Autodesk Inventor part; units mm, degrees
(part 2 of 2)
  spline S23 degree 3 poles (-70.3102, 10.593) (-70.1991, 10.6097) (-69.9769, 10.6432) (-69.6422, 10.6835) (-69.3067, 10.7162) (-68.9704, 10.7401) (-68.6336, 10.7549) (-68.2966, 10.7599) (-67.9595, 10.7543) (-67.6228, 10.7372) (-67.3429, 10.7123) (-67.1199, 10.6849) (-66.9531, 10.6603) (-66.787, 10.6316) (-66.6222, 10.5966) (-66.4851, 10.5659) (-66.3739, 10.5488) (-66.2901, 10.5406) (-66.2059, 10.536) (-66.1216, 10.5362) (-66.0374, 10.5419) (-65.9539, 10.5535) (-65.8715, 10.5716) (-65.7908, 10.5963) (-65.7126, 10.628) (-65.638, 10.6674) (-65.5675, 10.7136) (-65.501, 10.7656) (-65.4412, 10.8252) (-65.3876, 10.8903) (-65.3403, 10.9603) (-65.2902, 11.0611) (-65.2358, 11.1905) (-65.176, 11.3176) (-65.1345, 11.4222) (-65.1141, 11.5042) (-65.1017, 11.5876) (-65.0973, 11.6719) (-65.1031, 11.7561) (-65.1159, 11.8394) (-65.1366, 11.9213) (-65.1653, 12.0006) (-65.2008, 12.0771) (-65.2425, 12.1504) (-65.2898, 12.2203) (-65.3418, 12.2867) (-65.3981, 12.3495) (-65.4578, 12.4089) (-65.52, 12.4658) (-65.607, 12.537) (-65.7215, 12.6184) (-65.8578, 12.7175) (-65.9903, 12.8218) (-66.1201, 12.9293) (-66.2896, 13.0769) (-66.4953, 13.2682) (-66.7333, 13.5071) (-66.9629, 13.7539) (-67.1846, 14.0078) (-67.3988, 14.2681) (-67.606, 14.5341) (-67.8061, 14.8054) (-68, 15.0811) (-68.1237, 15.2687) (-68.1856, 15.3625) knots -1.078574 -1.078574 -1.078574 -1.078574 -1.044867 -1.011159 -0.977452 -0.943745 -0.910038 -0.876331 -0.842624 -0.808918 -0.775212 -0.758359 -0.741505 -0.724651 -0.707798 -0.690947 -0.68252 -0.674093 -0.665668 -0.657242 -0.648815 -0.640389 -0.631963 -0.623537 -0.61511 -0.606685 -0.598264 -0.589839 -0.581413 -0.57299 -0.564565 -0.556141 -0.539287 -0.522433 -0.514009 -0.505584 -0.49716 -0.488735 -0.48031 -0.471889 -0.463464 -0.455037 -0.446611 -0.438185 -0.429758 -0.421332 -0.412906 -0.40448 -0.396053 -0.387627 -0.370775 -0.353922 -0.337069 -0.320215 -0.303361 -0.269656 -0.235949 -0.202243 -0.168536 -0.134829 -0.101122 -0.067415 -0.033707 0 0 0 0 construction
  arc A27 (-67.448, 16.6395) -> (-68.1856, 15.3625) centre (-40.1144, 0) ccw construction
  spline S24 degree 3 poles (-67.448, 16.6395) (-67.3358, 16.6328) (-67.1115, 16.6194) (-66.7757, 16.5892) (-66.4407, 16.5514) (-66.1069, 16.5049) (-65.7744, 16.4494) (-65.4436, 16.3842) (-65.115, 16.3087) (-64.7893, 16.2219) (-64.5207, 16.1393) (-64.3082, 16.0662) (-64.1502, 16.0075) (-63.9937, 15.9448) (-63.8398, 15.8763) (-63.712, 15.8177) (-63.6069, 15.778) (-63.5265, 15.7525) (-63.4452, 15.7305) (-63.3627, 15.7131) (-63.2792, 15.7012) (-63.195, 15.6952) (-63.1107, 15.6957) (-63.0267, 15.7031) (-62.9436, 15.7179) (-62.8624, 15.7409) (-62.7838, 15.7715) (-62.708, 15.8085) (-62.6371, 15.8544) (-62.5711, 15.9069) (-62.5103, 15.9655) (-62.4404, 16.0537) (-62.3602, 16.169) (-62.2753, 16.2809) (-62.213, 16.3746) (-62.176, 16.4505) (-62.1464, 16.5295) (-62.1246, 16.6111) (-62.1128, 16.6946) (-62.108, 16.7788) (-62.1112, 16.8632) (-62.1228, 16.9467) (-62.1417, 17.029) (-62.1672, 17.1094) (-62.1989, 17.1875) (-62.236, 17.2633) (-62.2779, 17.3364) (-62.324, 17.407) (-62.373, 17.4756) (-62.4433, 17.5633) (-62.5384, 17.6667) (-62.6511, 17.792) (-62.759, 17.9215) (-62.8636, 18.0537) (-62.9988, 18.2332) (-63.1602, 18.4632) (-63.3433, 18.7463) (-63.5166, 19.0355) (-63.6806, 19.33) (-63.8361, 19.6291) (-63.9834, 19.9323) (-64.1227, 20.2393) (-64.2551, 20.5493) (-64.3371, 20.7586) (-64.3781, 20.8632) knots -1.078574 -1.078574 -1.078574 -1.078574 -1.044867 -1.011159 -0.977452 -0.943745 -0.910038 -0.876331 -0.842624 -0.808918 -0.775212 -0.758359 -0.741505 -0.724651 -0.707798 -0.690947 -0.68252 -0.674093 -0.665668 -0.657242 -0.648815 -0.640389 -0.631963 -0.623537 -0.61511 -0.606685 -0.598264 -0.589839 -0.581413 -0.57299 -0.564565 -0.556141 -0.539287 -0.522433 -0.514009 -0.505584 -0.49716 -0.488735 -0.48031 -0.471889 -0.463464 -0.455037 -0.446611 -0.438185 -0.429758 -0.421332 -0.412906 -0.40448 -0.396053 -0.387627 -0.370775 -0.353922 -0.337069 -0.320215 -0.303361 -0.269656 -0.235949 -0.202243 -0.168536 -0.134829 -0.101122 -0.067415 -0.033707 0 0 0 0 construction
  arc A28 (-63.3911, 21.9589) -> (-64.3781, 20.8632) centre (-40.1144, 0) ccw construction
  spline S25 degree 3 poles (-63.3911, 21.9589) (-63.2828, 21.929) (-63.0662, 21.8693) (-62.744, 21.7699) (-62.4242, 21.6633) (-62.1073, 21.5484) (-61.7936, 21.4249) (-61.4836, 21.2924) (-61.178, 21.1502) (-60.8773, 20.9976) (-60.6318, 20.861) (-60.4392, 20.7453) (-60.2968, 20.655) (-60.1568, 20.5612) (-60.0204, 20.4621) (-59.9077, 20.3783) (-59.8131, 20.3175) (-59.7398, 20.276) (-59.6648, 20.2375) (-59.5877, 20.2034) (-59.5085, 20.1743) (-59.4275, 20.151) (-59.3448, 20.134) (-59.2611, 20.1237) (-59.1768, 20.1209) (-59.0926, 20.1265) (-59.0093, 20.1401) (-58.9275, 20.1605) (-58.8486, 20.1907) (-58.7731, 20.2283) (-58.7014, 20.273) (-58.6147, 20.3447) (-58.5124, 20.4409) (-58.406, 20.5326) (-58.3256, 20.6113) (-58.2736, 20.6779) (-58.2283, 20.749) (-58.19, 20.8243) (-58.1611, 20.9036) (-58.1389, 20.9849) (-58.1245, 21.0681) (-58.1184, 21.1522) (-58.1198, 21.2366) (-58.1281, 21.3205) (-58.1428, 21.4036) (-58.1633, 21.4854) (-58.1892, 21.5656) (-58.2196, 21.6442) (-58.2532, 21.7215) (-58.3038, 21.8219) (-58.3753, 21.9429) (-58.4595, 22.0889) (-58.5381, 22.238) (-58.6129, 22.389) (-58.7078, 22.5927) (-58.8179, 22.8512) (-58.9381, 23.1662) (-59.0475, 23.4851) (-59.1467, 23.8073) (-59.2366, 24.1322) (-59.3177, 24.4594) (-59.3901, 24.7886) (-59.4551, 25.1194) (-59.4918, 25.3411) (-59.5102, 25.452) knots -1.078574 -1.078574 -1.078574 -1.078574 -1.044867 -1.011159 -0.977452 -0.943745 -0.910038 -0.876331 -0.842624 -0.808918 -0.775212 -0.758359 -0.741505 -0.724651 -0.707798 -0.690947 -0.68252 -0.674093 -0.665668 -0.657242 -0.648815 -0.640389 -0.631963 -0.623537 -0.61511 -0.606685 -0.598264 -0.589839 -0.581413 -0.57299 -0.564565 -0.556141 -0.539287 -0.522433 -0.514009 -0.505584 -0.49716 -0.488735 -0.48031 -0.471889 -0.463464 -0.455037 -0.446611 -0.438185 -0.429758 -0.421332 -0.412906 -0.40448 -0.396053 -0.387627 -0.370775 -0.353922 -0.337069 -0.320215 -0.303361 -0.269656 -0.235949 -0.202243 -0.168536 -0.134829 -0.101122 -0.067415 -0.033707 0 0 0 0 construction
  arc A29 (-58.3169, 26.3186) -> (-59.5102, 25.452) centre (-40.1144, 0) ccw construction
  spline S26 degree 3 poles (-58.3169, 26.3186) (-58.2172, 26.2668) (-58.0177, 26.1633) (-57.7233, 25.9992) (-57.4326, 25.8284) (-57.1465, 25.6501) (-56.8654, 25.4641) (-56.5897, 25.27) (-56.3203, 25.0674) (-56.058, 24.8556) (-55.8462, 24.6709) (-55.6818, 24.5177) (-55.5614, 24.3998) (-55.4439, 24.2789) (-55.3311, 24.1537) (-55.2383, 24.0483) (-55.1584, 23.9691) (-55.0953, 23.9132) (-55.03, 23.86) (-54.9616, 23.8106) (-54.8902, 23.7657) (-54.8158, 23.7261) (-54.7385, 23.6922) (-54.6587, 23.6648) (-54.5768, 23.6445) (-54.4933, 23.6325) (-54.4091, 23.6284) (-54.3247, 23.6314) (-54.2413, 23.6446) (-54.1597, 23.6656) (-54.0803, 23.6945) (-53.9805, 23.7466) (-53.8604, 23.8194) (-53.7373, 23.887) (-53.6423, 23.9472) (-53.5776, 24.0015) (-53.5185, 24.0617) (-53.4654, 24.1273) (-53.4206, 24.1989) (-53.382, 24.2738) (-53.3506, 24.3522) (-53.3272, 24.4332) (-53.311, 24.516) (-53.3016, 24.5999) (-53.2988, 24.6842) (-53.3019, 24.7684) (-53.3105, 24.8523) (-53.3238, 24.9355) (-53.3407, 25.0181) (-53.3692, 25.1269) (-53.414, 25.26) (-53.4661, 25.4203) (-53.5119, 25.5825) (-53.5538, 25.7458) (-53.6042, 25.9648) (-53.6582, 26.2405) (-53.7103, 26.5736) (-53.7509, 26.9083) (-53.781, 27.2441) (-53.8014, 27.5806) (-53.8126, 27.9175) (-53.8151, 28.2546) (-53.8099, 28.5917) (-53.7997, 28.8161) (-53.7946, 28.9284) knots -1.078574 -1.078574 -1.078574 -1.078574 -1.044867 -1.011159 -0.977452 -0.943745 -0.910038 -0.876331 -0.842624 -0.808918 -0.775212 -0.758359 -0.741505 -0.724651 -0.707798 -0.690947 -0.68252 -0.674093 -0.665668 -0.657242 -0.648815 -0.640389 -0.631963 -0.623537 -0.61511 -0.606685 -0.598264 -0.589839 -0.581413 -0.57299 -0.564565 -0.556141 -0.539287 -0.522433 -0.514009 -0.505584 -0.49716 -0.488735 -0.48031 -0.471889 -0.463464 -0.455037 -0.446611 -0.438185 -0.429758 -0.421332 -0.412906 -0.40448 -0.396053 -0.387627 -0.370775 -0.353922 -0.337069 -0.320215 -0.303361 -0.269656 -0.235949 -0.202243 -0.168536 -0.134829 -0.101122 -0.067415 -0.033707 0 0 0 0 construction
  arc A30 (-52.4472, 29.528) -> (-53.7946, 28.9284) centre (-40.1144, 0) ccw construction
  spline S27 degree 3 poles (-52.4472, 29.528) (-52.3604, 29.4566) (-52.1868, 29.3139) (-51.933, 29.0921) (-51.6842, 28.8647) (-51.4414, 28.6308) (-51.205, 28.3904) (-50.9758, 28.1432) (-50.7543, 27.889) (-50.5418, 27.6273) (-50.3731, 27.4026) (-50.2441, 27.2186) (-50.1508, 27.0782) (-50.061, 26.9355) (-49.9768, 26.7896) (-49.9078, 26.6672) (-49.8462, 26.5732) (-49.7961, 26.5054) (-49.7432, 26.4397) (-49.6867, 26.3772) (-49.6261, 26.3185) (-49.5616, 26.2642) (-49.4931, 26.215) (-49.4207, 26.1716) (-49.3448, 26.1347) (-49.2656, 26.1056) (-49.1841, 26.0841) (-49.101, 26.0695) (-49.0166, 26.065) (-48.9324, 26.0687) (-48.8487, 26.0804) (-48.7403, 26.1106) (-48.6077, 26.1568) (-48.4732, 26.1973) (-48.3678, 26.2365) (-48.2932, 26.2762) (-48.2229, 26.3228) (-48.1573, 26.3759) (-48.0986, 26.4366) (-48.0452, 26.5019) (-47.9983, 26.572) (-47.9585, 26.6464) (-47.9255, 26.724) (-47.8989, 26.8041) (-47.8785, 26.8859) (-47.864, 26.969) (-47.855, 27.0528) (-47.8508, 27.137) (-47.8501, 27.2213) (-47.8554, 27.3336) (-47.8716, 27.4732) (-47.8891, 27.6408) (-47.9003, 27.809) (-47.9072, 27.9774) (-47.911, 28.2021) (-47.9065, 28.483) (-47.8882, 28.8197) (-47.8584, 29.1555) (-47.818, 29.4902) (-47.768, 29.8235) (-47.7089, 30.1554) (-47.6412, 30.4857) (-47.5661, 30.8143) (-47.5094, 31.0318) (-47.4811, 31.1405) knots -1.078574 -1.078574 -1.078574 -1.078574 -1.044867 -1.011159 -0.977452 -0.943745 -0.910038 -0.876331 -0.842624 -0.808918 -0.775212 -0.758359 -0.741505 -0.724651 -0.707798 -0.690947 -0.68252 -0.674093 -0.665668 -0.657242 -0.648815 -0.640389 -0.631963 -0.623537 -0.61511 -0.606685 -0.598264 -0.589839 -0.581413 -0.57299 -0.564565 -0.556141 -0.539287 -0.522433 -0.514009 -0.505584 -0.49716 -0.488735 -0.48031 -0.471889 -0.463464 -0.455037 -0.446611 -0.438185 -0.429758 -0.421332 -0.412906 -0.40448 -0.396053 -0.387627 -0.370775 -0.353922 -0.337069 -0.320215 -0.303361 -0.269656 -0.235949 -0.202243 -0.168536 -0.134829 -0.101122 -0.067415 -0.033707 0 0 0 0 construction
  arc A31 (-46.0385, 31.4469) -> (-47.4811, 31.1405) centre (-40.1144, 0) ccw construction
  spline S28 degree 3 poles (-46.0385, 31.4469) (-45.9685, 31.359) (-45.8283, 31.1833) (-45.6261, 30.9136) (-45.43, 30.6394) (-45.2412, 30.3601) (-45.06, 30.0759) (-44.8871, 29.7864) (-44.7234, 29.4917) (-44.5699, 29.1916) (-44.4516, 28.9367) (-44.3637, 28.7299) (-44.3016, 28.5732) (-44.2435, 28.415) (-44.1914, 28.2547) (-44.1494, 28.1206) (-44.1086, 28.0159) (-44.0738, 27.9391) (-44.0357, 27.8639) (-43.9934, 27.791) (-43.9464, 27.721) (-43.8945, 27.6544) (-43.8377, 27.5921) (-43.776, 27.5346) (-43.7094, 27.4828) (-43.638, 27.4378) (-43.5627, 27.3998) (-43.4844, 27.3683) (-43.4029, 27.3463) (-43.3197, 27.3324) (-43.2354, 27.3264) (-43.1231, 27.3335) (-42.9838, 27.3511) (-42.8439, 27.3628) (-42.7325, 27.3792) (-42.6513, 27.4025) (-42.5729, 27.4334) (-42.4977, 27.4718) (-42.4277, 27.5189) (-42.3619, 27.5717) (-42.3014, 27.6305) (-42.247, 27.695) (-42.1985, 27.7641) (-42.1559, 27.8368) (-42.119, 27.9127) (-42.0875, 27.9909) (-42.0612, 28.071) (-42.0396, 28.1525) (-42.0214, 28.2348) (-42.0033, 28.3458) (-41.9901, 28.4856) (-41.9724, 28.6532) (-41.9483, 28.8201) (-41.9201, 28.9863) (-41.8771, 29.2068) (-41.8143, 29.4807) (-41.7264, 29.8062) (-41.6274, 30.1284) (-41.5183, 30.4474) (-41.4001, 30.7631) (-41.2733, 31.0755) (-41.1384, 31.3844) (-40.9966, 31.6902) (-40.8959, 31.8912) (-40.8456, 31.9916) knots -1.078574 -1.078574 -1.078574 -1.078574 -1.044867 -1.011159 -0.977452 -0.943745 -0.910038 -0.876331 -0.842624 -0.808918 -0.775212 -0.758359 -0.741505 -0.724651 -0.707798 -0.690947 -0.68252 -0.674093 -0.665668 -0.657242 -0.648815 -0.640389 -0.631963 -0.623537 -0.61511 -0.606685 -0.598264 -0.589839 -0.581413 -0.57299 -0.564565 -0.556141 -0.539287 -0.522433 -0.514009 -0.505584 -0.49716 -0.488735 -0.48031 -0.471889 -0.463464 -0.455037 -0.446611 -0.438185 -0.429758 -0.421332 -0.412906 -0.40448 -0.396053 -0.387627 -0.370775 -0.353922 -0.337069 -0.320215 -0.303361 -0.269656 -0.235949 -0.202243 -0.168536 -0.134829 -0.101122 -0.067415 -0.033707 0 0 0 0 construction
  arc A32 (-39.3709, 31.9914) -> (-40.8456, 31.9916) centre (-40.1144, 0) ccw construction
  spline S29 degree 3 poles (-39.3709, 31.9914) (-39.3206, 31.8909) (-39.2201, 31.6899) (-39.0784, 31.384) (-38.9436, 31.075) (-38.8169, 30.7626) (-38.6988, 30.4469) (-38.5899, 30.1278) (-38.491, 29.8055) (-38.4032, 29.48) (-38.3405, 29.2061) (-38.2976, 28.9856) (-38.2694, 28.8194) (-38.2454, 28.6525) (-38.2278, 28.4849) (-38.2146, 28.345) (-38.1965, 28.2341) (-38.1784, 28.1518) (-38.1568, 28.0703) (-38.1305, 27.9902) (-38.0991, 27.9119) (-38.0622, 27.8361) (-38.0196, 27.7633) (-37.9712, 27.6942) (-37.9168, 27.6296) (-37.8563, 27.5708) (-37.7906, 27.518) (-37.7206, 27.4709) (-37.6454, 27.4325) (-37.5669, 27.4015) (-37.4858, 27.3782) (-37.3744, 27.3617) (-37.2345, 27.35) (-37.0952, 27.3323) (-36.9829, 27.3252) (-36.8986, 27.3311) (-36.8154, 27.3451) (-36.7339, 27.367) (-36.6556, 27.3985) (-36.5803, 27.4364) (-36.5089, 27.4814) (-36.4423, 27.5332) (-36.3805, 27.5907) (-36.3237, 27.653) (-36.2718, 27.7195) (-36.2248, 27.7895) (-36.1824, 27.8624) (-36.1443, 27.9376) (-36.1094, 28.0143) (-36.0686, 28.1191) (-36.0266, 28.2531) (-35.9744, 28.4134) (-35.9162, 28.5716) (-35.8541, 28.7283) (-35.7661, 28.9351) (-35.6477, 29.1899) (-35.4941, 29.49) (-35.3303, 29.7846) (-35.1573, 30.074) (-34.976, 30.3582) (-34.787, 30.6373) (-34.5908, 30.9115) (-34.3885, 31.1811) (-34.2483, 31.3568) (-34.1782, 31.4446) knots -1.078574 -1.078574 -1.078574 -1.078574 -1.044867 -1.011159 -0.977452 -0.943745 -0.910038 -0.876331 -0.842624 -0.808918 -0.775212 -0.758359 -0.741505 -0.724651 -0.707798 -0.690947 -0.68252 -0.674093 -0.665668 -0.657242 -0.648815 -0.640389 -0.631963 -0.623537 -0.61511 -0.606685 -0.598264 -0.589839 -0.581413 -0.57299 -0.564565 -0.556141 -0.539287 -0.522433 -0.514009 -0.505584 -0.49716 -0.488735 -0.48031 -0.471889 -0.463464 -0.455037 -0.446611 -0.438185 -0.429758 -0.421332 -0.412906 -0.40448 -0.396053 -0.387627 -0.370775 -0.353922 -0.337069 -0.320215 -0.303361 -0.269656 -0.235949 -0.202243 -0.168536 -0.134829 -0.101122 -0.067415 -0.033707 0 0 0 0 construction
  arc A33 (-32.7358, 31.1377) -> (-34.1782, 31.4446) centre (-40.1144, 0) ccw construction
  circle A34 centre (-40.1144, 0) radius 6.16 projected
  line L6 (-57.3551, -17.4071) -> (-47.0575, -5.9749) construction
  arc A35 (-48.8864, 2.6377) -> (-47.0575, -5.9749) centre (-40.1144, 0) ccw construction
  line L7 (-48.8864, 2.6377) -> (-62.9413, 8.8985) construction
  arc A36 (-62.9413, 8.8985) -> (-57.3551, -17.4071) centre (-40.1144, 0) ccw construction
  line L8 (-28.8869, -21.776) -> (-36.5775, -8.4496) construction
  arc A37 (-45.3337, -7.5276) -> (-36.5775, -8.4496) centre (-40.1144, 0) ccw construction
  line L9 (-45.3337, -7.5276) -> (-55.6313, -18.9599) construction
  arc A38 (-55.6313, -18.9599) -> (-28.8869, -21.776) centre (-40.1144, 0) ccw construction
  line L10 (-36.398, 24.2165) -> (-38.0093, 8.9148) construction
  arc A39 (-31.4673, 3.0221) -> (-38.0093, 8.9148) centre (-40.1144, 0) ccw construction
  line L11 (-31.4673, 3.0221) -> (-16.4166, 6.2182) construction
  arc A40 (-16.4166, 6.2182) -> (-36.398, 24.2165) centre (-40.1144, 0) ccw construction
  line L12 (-40.3165, 9.1578) -> (-38.7053, 24.4594) construction
  arc A41 (-38.7053, 24.4594) -> (-61.9972, 11.0178) centre (-40.1144, 0) ccw construction
  line L13 (-61.9972, 11.0178) -> (-47.9424, 4.7569) construction
  arc A42 (-40.3165, 9.1578) -> (-47.9424, 4.7569) centre (-40.1144, 0) ccw construction
  line L14 (-15.9347, 3.9489) -> (-30.9854, 0.7527) construction
  arc A43 (-34.5681, -7.29) -> (-30.9854, 0.7527) centre (-40.1144, 0) ccw construction
  line L15 (-34.5681, -7.29) -> (-26.8775, -20.6164) construction
  arc A44 (-26.8775, -20.6164) -> (-15.9347, 3.9489) centre (-40.1144, 0) ccw construction
  line L16 (12.8712, -37.5) -> (-72.1144, -37.5)
  line L17 (-72.1144, -37.5) -> (-72.1144, -42.5)
  line L18 (-72.1144, -42.5) -> (12.8712, -42.5)
  line L19 (12.8712, -42.5) -> (12.8712, -37.5)
  line L20 (7.4686, 10.6) -> (-7.6974, 10.6)
  arc A45 (-7.6974, 10.6) -> (-7.6974, -10.6) centre (0, 0) ccw
  line L21 (-7.6974, -10.6) -> (7.4686, -10.6)
  arc A46 (7.4686, -10.6) -> (7.4686, 10.6) centre (-0.2288, 0) ccw
  line L22 (12.7943, 1.4177) -> (9.7712, 1.4177)
  line L23 (-10, 1.4177) -> (-13.0231, 1.4177)
  line L24 (12.8712, 0) -> (12.8712, -37.5)
  line L25 (-13.1, 0) -> (-13.1, -37.5)
  circle A47 centre (-40.1144, 0) radius 32 construction
  circle A48 centre (-40.1144, 0) radius 9.16
  line L26 (-28.8869, 0) -> (-51.3564, 0) construction
  line L27 (-33.9544, 0) -> (-33.9544, 10.593)
  line L28 (-46.2744, 0) -> (-46.2744, 10.593)
  line L29 (-30.9544, 0) -> (-30.9544, -37.5)
  line L30 (-49.2744, 0) -> (-49.2744, -37.5)
  point P0 (24.8534, -22.5561)
  point P1 (-33.9544, 6.7794)
  point P2 (-46.2744, 6.7794)
  dimension "d0" = 0.1
  dimension "d1" = 5
  dimension "d2" = 5.5
  dimension "d3" = 3
  dimension "d9" = 3
  constraints: 38 end point, 24 point on circle, 12 point on line, 9 tangent, 8 centre point, 7 perpendicular, 3 vertical, 2 horizontal, 2 parallel, 1 coincident, 1 collinear, 1 concentric, 8 other
  measures "d0" radial gap between concentric circles of A0 A3
  measures "d1" distance of L16.end L17.end
  measures "d2" distance edge to line of A17 L16
  measures "d3" radial gap between concentric circles of A3 A46
  measures "d9" radial gap between concentric circles of A34 A48
extrude "Extrusion1" add sketch "Sketch1" against normal blind 10 contours L22 A46 L21 A45 L23 A2 L3 A3 | L24 L16 L25 A45 L21 A46 | L19 L18 L17 L16 | L16 L30 A48 L29 | A48 L28 A34 L27 picked at (-46.6973, 4.0461)
extrude "Extrusion2" add sketch "Sketch1" along normal up to surface (14.28 mm away) contours L19 L18 L17 L16
fillet "Fillet1" radius 5.75 2 edges at (12.0591, 23.9738, 27.06) (37.8764, 23.9738, 27.06)
mirror "Mirror2" about plane through (24.9677, 22.5561, 7.78) normal (0, 0, 1) of "Extrusion1", "Extrusion2"
sketch "Sketch2" plane through (96.9677, -19.9439, 32.06) normal (1, 0, 0) x (0, 0, -1)
  line L0 (32.06, 5) -> (32.06, 14.3934) construction
  line L1 (32.06, 14.3934) -> (27.06, 14.3934) construction
  line L2 (27.06, 5) -> (27.06, 14.3934) construction
  line L3 (32.06, 5) -> (27.06, 5) construction
  line L4 (26.56, 4.5) -> (26.56, 14.8934)
  line L5 (26.56, 14.8934) -> (32.56, 14.8934) construction
  line L6 (32.56, 14.8934) -> (32.56, 4.5) construction
  line L7 (32.56, 4.5) -> (26.56, 4.5) construction
  line L8 (26.56, 5) -> (23.56, 5)
  line L9 (23.56, 5) -> (23.56, 14.3934)
  line L10 (23.56, 14.3934) -> (26.56, 14.3934)
  line L11 (26.56, 14.3934) -> (26.56, 5) construction
  line L12 (38.56, 5) -> (10, 5) projected
  line L13 (32.56, 5) -> (35.56, 5)
  line L14 (35.56, 5) -> (35.56, 14.3934)
  line L15 (35.56, 14.3934) -> (32.56, 14.3934)
  line L16 (32.56, 14.3934) -> (32.56, 5)
  point P0 (32.06, 19.9439)
  dimension "d10" = 0.5
  dimension "d11" = 3
  dimension "d12" = 3
  constraints: 24 end point, 4 parallel, 3 point on line, 2 horizontal, 2 perpendicular, 3 other
  measures "d10" distance between parallel lines of L3 L7
  measures "d11" distance of L9.end L10.end
  measures "d12" distance of L15.end L14.end
extrude "Extrusion3" add sketch "Sketch2" against normal up to surface (84.9856 mm away)
body "Solid1"
